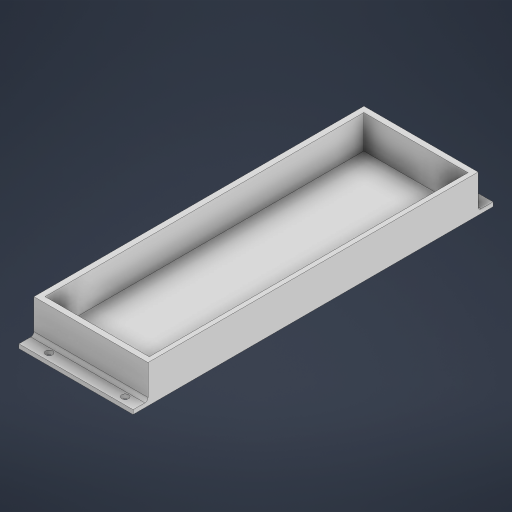
# Autodesk Inventor part: beban
Saved by Autodesk Inventor 2024.3 (Build 283343000, 343)
## iProperties
Created: 2025-06-23
Part Number: beban
Material: Generic
Document SubType Name: Modeling
Designer: Akbar Syihabuddin
Density: 1 g/cm^3
Appearance: Default
Author: Akbar Syihabuddin
Autodesk Inventor part; units mm, degrees
ref_plane "YZ Plane" through (0, 0, 0) normal (1, 0, 0) x (0, 1, 0)
ref_plane "XZ Plane" through (0, 0, 0) normal (0, 1, 0) x (-1, 0, 0)
ref_plane "XY Plane" through (0, 0, 0) normal (0, 0, 1) x (1, 0, 0)
sketch "Sketch1" plane through (0, 0, 0) normal (0, 1, 0) x (-1, 0, 0)
  line L0 (40.5829, -68.5109) -> (-9.4171, -68.5109)
  line L1 (-9.4171, -68.5109) -> (-9.4171, 7.9891)
  line L2 (-9.4171, 7.9891) -> (40.5829, 7.9891)
  line L3 (40.5829, 7.9891) -> (40.5829, -68.5109)
  line L4 (40.5829, -68.5109) -> (-9.4171, -68.5109)
  line L5 (-9.4171, -68.5109) -> (-9.4171, -145.0109)
  line L6 (-9.4171, -145.0109) -> (40.5829, -145.0109)
  line L7 (40.5829, -145.0109) -> (40.5829, -68.5109)
  line L8 (43.2164, 17.8584) -> (43.2164, -154.8803)
  line L9 (43.2164, -68.5109) -> (-11.5522, -68.5109)
  line L10 (-11.5522, -68.5109) -> (-11.5522, -147.7105)
  line L11 (-11.5522, -147.7105) -> (43.2164, -147.7105)
  line L12 (43.2164, -147.7105) -> (43.2164, -68.5109)
  line L13 (-11.5522, 10.6887) -> (43.2164, 10.6887)
  line L14 (-11.5522, -68.5109) -> (-11.5522, 10.6887)
  circle A0 centre (-4.2663, -151.3765) radius 1.65
  circle A1 centre (32.2203, -151.3765) radius 1.65
  line L15 (43.2164, -147.7105) -> (43.2164, -154.8803)
  line L16 (43.2164, -154.8803) -> (-11.5522, -154.8803)
  line L17 (-13.2912, -151.8803) -> (16.3367, -151.8803)
  line L18 (-11.5522, -154.8803) -> (-11.5522, -147.7105)
  line L19 (-11.5522, 10.6887) -> (43.2164, 10.6887)
  line L20 (-13.2912, 14.8584) -> (16.3367, 14.8584)
  circle A2 centre (-4.2663, 14.3547) radius 1.65
  line L21 (-11.5522, 17.8584) -> (-11.5522, 10.6887)
  line L22 (43.2164, 17.8584) -> (-11.5522, 17.8584)
  circle A3 centre (32.2203, 14.3547) radius 1.65
  line L23 (43.2164, 10.6887) -> (43.2164, 17.8584)
  point P0 (0, 0)
  point P1 (7.1317, -61.1506)
  point P2 (-9.4171, -68.5109)
  dimension "d2" = 50
  dimension "d3" = 76.5
  dimension "d4" = 76.5
  dimension "d5" = 3.3
  dimension "d6" = 3.3
  constraints: 48 end point, 7 parallel, 7 symmetric about line, 4 centre point, 4 perpendicular, 3 horizontal, 1 collinear, 1 midpoint, 1 vertical, 2 other
  measures "d2" distance of L1.end L2.end
  measures "d3" distance of L0.end L1.end
  measures "d4" distance of L5.end L4.end
  measures "d5" diameter of A0
  measures "d6" diameter of A1
extrude "Extrusion1" add sketch "Sketch1" along normal blind 18 contours L9 L8 L11 L10 L5 L6 L7 | L3 L2 L1 L9 L14 L13 L8
extrude "Extrusion2" add sketch "Sketch1" along normal blind 2 contours L7 L6 L5 L0 | L0 L1 L2 L3 | L13 L21 L22 L8 | L8 L16 L18 L11
fillet "Fillet1" radius 1.5 1 edges at (-15.8321, 2, -147.7105)
fillet "Fillet2" radius 1.5 1 edges at (-15.8321, 2, 10.6887)
body "Solid1"
